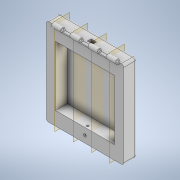
# Autodesk Inventor part: Bottom
Saved by Autodesk Inventor 2022 (Build 260153000, 153)
## iProperties
Created: 2022-03-05
Part Number: Bottom
Material: Generic
Document SubType Name: Modeling
Designer: Stump
Density: 1 g/cm^3
Appearance: Default
Author: Stump
Autodesk Inventor part; units mm, degrees
ref_plane "XZ Plane" through (0, 0, 0) normal (0, 1, 0) x (-1, 0, 0)
ref_plane "XY Plane" through (0, 0, 0) normal (0, 0, 1) x (1, 0, 0)
sketch "Sketch1" plane through (0, 0, 0) normal (0, 0, 1) x (1, 0, 0)
  line L0 (0, 0) -> (165.2524, 0)
  line L1 (165.2524, 0) -> (165.2524, 167.64)
  line L2 (165.2524, 167.64) -> (0, 167.64)
  line L3 (0, 167.64) -> (0, 0)
  line L4 (82.6262, 167.64) -> (82.6262, 205.74) construction
  line L5 (82.6262, 0) -> (82.6262, -38.1) construction
  line L6 (0, 83.82) -> (-25.4, 83.82) construction
  line L7 (165.2524, 83.82) -> (190.6524, 83.82) construction
  line L8 (-25.4981, -38.1) -> (190.6088, -38.1)
  line L9 (190.6088, -38.1) -> (190.6088, 205.74)
  line L10 (190.6088, 205.74) -> (-25.4981, 205.74)
  line L11 (-25.4981, 205.74) -> (-25.4981, -38.1)
  dimension "d0" = 165.2524
  dimension "d1" = 167.64
  dimension "d2" = 38.1
  dimension "d3" = 38.1
  dimension "d4" = 25.4
  dimension "d5" = 25.4
  constraints: 24 end point, 4 horizontal, 4 midpoint, 4 parallel, 2 perpendicular, 2 vertical
  measures "d0" distance of L2.end L1.end
  measures "d1" distance of L1.end L0.end
  measures "d2" distance of L4.start L4.end
  measures "d3" distance of L5.start L5.end
  measures "d4" distance of L6.start L6.end
  measures "d5" distance of L7.start L7.end
extrude "Extrusion1" add sketch "Sketch1" along normal blind 37.592
sketch "Sketch3" plane through (0, 0, 0) normal (0, 0, -1) x (-1, 0, 0)
  line L0 (6.0775, -8.2655) -> (-172.3593, -8.2655)
  line L1 (-172.3593, -8.2655) -> (-172.3593, 173.0886)
  line L2 (-172.3593, 173.0886) -> (6.0775, 173.0886)
  line L3 (6.0775, 173.0886) -> (6.0775, -8.2655)
  point P0 (0, 0)
  constraints: 8 end point, 2 parallel, 1 horizontal, 1 perpendicular
extrude "Extrusion3" add sketch "Sketch3" against normal blind 4.699
fillet "Fillet1" radius 6.35 8 edges at (-25.4981, 205.74, 18.796) (-25.4981, -38.1, 18.796) (190.6088, -38.1, 18.796) (190.6088, 205.74, 18.796) (190.6088, 83.82, 0) (82.5553, -38.1, 0) (-25.4981, 83.82, 0) (82.5553, 205.74, 0)
ref_plane "Work Plane1" through (0.254, 0, 0) normal (1, 0, 0) x (0, 1, 0)
sketch "Sketch4" plane through (0.254, 0, 0) normal (1, 0, 0) x (0, 1, 0)
  line L0 (205.74, 37.592) -> (217.17, 37.592) construction
  line L1 (217.17, 37.592) -> (217.17, 49.022) construction
  line L2 (217.17, 49.022) -> (205.74, 49.022) construction
  line L3 (205.74, 49.022) -> (205.74, 37.592) construction
  circle A0 centre (211.455, 43.307) radius 5.715
  circle A1 centre (211.455, 43.307) radius 3.302
  point P0 (0, 0)
  dimension "d14" = 11.43
  dimension "d15" = 11.43
  dimension "d16" = 6.604
  constraints: 8 end point, 3 perpendicular, 2 centre point, 1 coincident, 1 horizontal, 1 tangent
  measures "d14" distance of L0.start L0.end
  measures "d15" distance of L0.end L1.end
  measures "d16" diameter of A1
extrude "Extrusion4" add sketch "Sketch4" along normal blind 25.4
ref_plane "Work Plane2" through (51.308, 0, 0) normal (1, 0, 0) x (0, 1, 0)
sketch "Sketch5" plane through (51.308, 0, 0) normal (1, 0, 0) x (0, 1, 0)
  line L0 (205.74, 37.592) -> (217.17, 37.592) construction
  line L1 (217.17, 37.592) -> (217.17, 49.022) construction
  circle A0 centre (211.455, 43.307) radius 5.715
  circle A1 centre (211.455, 43.307) radius 3.302
  point P0 (0, 0)
  dimension "d20" = 11.43
  dimension "d21" = 11.43
  dimension "d22" = 6.604
  constraints: 4 end point, 2 centre point, 1 coincident, 1 horizontal, 1 perpendicular
  measures "d20" distance of L0.start L0.end
  measures "d21" distance of L0.end L1.end
  measures "d22" diameter of A1
extrude "Extrusion5" add sketch "Sketch5" along normal blind 25.4
ref_plane "Work Plane3" through (102.362, 0, 0) normal (1, 0, 0) x (0, 1, 0)
sketch "Sketch6" plane through (102.362, 0, 0) normal (1, 0, 0) x (0, 1, 0)
  line L0 (205.74, 37.592) -> (217.17, 37.592) construction
  line L1 (217.17, 37.592) -> (217.17, 49.022) construction
  circle A0 centre (211.455, 43.307) radius 5.715
  circle A1 centre (211.455, 43.307) radius 3.302
  point P0 (0, 0)
  dimension "d26" = 11.43
  dimension "d27" = 11.43
  dimension "d28" = 6.604
  constraints: 4 end point, 2 centre point, 1 coincident, 1 horizontal, 1 perpendicular
  measures "d26" distance of L0.start L0.end
  measures "d27" distance of L0.end L1.end
  measures "d28" diameter of A1
extrude "Extrusion6" add sketch "Sketch6" along normal blind 25.4
ref_plane "Work Plane4" through (153.416, 0, 0) normal (1, 0, 0) x (0, 1, 0)
sketch "Sketch7" plane through (153.416, 0, 0) normal (1, 0, 0) x (0, 1, 0)
  line L0 (205.74, 37.592) -> (217.17, 37.592) construction
  line L1 (217.17, 37.592) -> (217.17, 49.022) construction
  circle A0 centre (211.455, 43.307) radius 5.715
  circle A1 centre (211.455, 43.307) radius 3.302
  point P0 (0, 0)
  dimension "d32" = 11.43
  dimension "d33" = 11.43
  dimension "d34" = 6.604
  constraints: 4 end point, 2 centre point, 1 coincident, 1 horizontal, 1 perpendicular
  measures "d32" distance of L0.start L0.end
  measures "d33" distance of L0.end L1.end
  measures "d34" diameter of A1
extrude "Extrusion7" add sketch "Sketch7" along normal blind 25.4
sketch "Sketch9" plane through (0.254, 0, 0) normal (1, 0, 0) x (0, 1, 0)
  line L0 (199.39, 37.592) -> (199.39, 6.35) projected
  line L1 (207.6697, 43.307) -> (199.39, 43.307)
  line L2 (199.39, 43.307) -> (199.39, 35.6964)
  line L3 (199.39, 35.6964) -> (207.6697, 35.6964)
  line L4 (207.6697, 39.5017) -> (207.6697, 43.307)
  line L5 (199.39, 35.6964) -> (211.3726, 35.6964)
  line L6 (211.3726, 35.6964) -> (211.3726, 39.5017)
  line L7 (211.3726, 39.5017) -> (207.6697, 39.5017)
  line L8 (199.39, 39.5017) -> (199.39, 35.6964)
  point P0 (0, 0)
  point P1 (199.39, 37.592)
  constraints: 16 end point, 4 parallel, 2 horizontal, 2 perpendicular, 1 point on line
extrude "Extrusion8" add sketch "Sketch9" along normal blind 178.562
sketch "Sketch10" plane through (0.254, 211.3726, 35.6964) normal (0, 1, 0) x (1, 0, 0)
  line L0 (102.108, -1.8961) -> (102.108, -3.8053) projected
  line L1 (127.508, -1.8961) -> (102.108, -1.8961) projected
  line L2 (127.508, -3.8053) -> (127.508, -1.8961) projected
  line L3 (127.508, -3.8053) -> (153.162, -3.8053) projected
  line L4 (153.162, -1.8961) -> (153.162, -3.8053) projected
  line L5 (178.562, -1.8961) -> (153.162, -1.8961) projected
  line L6 (178.562, 0) -> (178.562, -1.8961) projected
  line L7 (0, 0) -> (178.562, 0) projected
  line L8 (0, 0) -> (0, -1.8961) projected
  line L9 (25.4, -1.8961) -> (0, -1.8961) projected
  line L10 (25.4, -3.8053) -> (25.4, -1.8961) projected
  line L11 (25.4, -3.8053) -> (51.054, -3.8053) projected
  line L12 (51.054, -1.8961) -> (51.054, -3.8053) projected
  line L13 (76.454, -1.8961) -> (51.054, -1.8961) projected
  line L14 (76.454, -3.8053) -> (76.454, -1.8961) projected
  line L15 (76.454, -3.8053) -> (102.108, -3.8053) projected
  line L16 (0, 0) -> (178.562, 0) projected
  line L17 (0, -7.6106) -> (178.562, -7.6106) projected
  line L18 (153.162, 0) -> (127.508, 0)
  line L19 (127.508, 0) -> (127.508, -7.6106)
  line L20 (127.508, -7.6106) -> (153.162, -7.6106)
  line L21 (153.162, -7.6106) -> (153.162, 0)
  line L22 (76.454, -7.6106) -> (102.108, -7.6106) projected
  line L23 (102.108, 0) -> (76.454, 0)
  line L24 (76.454, 0) -> (76.454, -7.6106)
  line L25 (76.454, -7.6106) -> (102.108, -7.6106)
  line L26 (102.108, -7.6106) -> (102.108, 0)
  line L27 (51.054, 0) -> (25.4, 0)
  line L28 (25.4, 0) -> (25.4, -7.6106)
  line L29 (25.4, -7.6106) -> (51.054, -7.6106)
  line L30 (51.054, -7.6106) -> (51.054, 0)
  point P0 (-0.254, 35.6964)
  point P1 (25.4, 0)
  point P2 (51.054, -7.6106)
  point P3 (51.054, -3.8053)
  point P4 (76.454, 0)
  constraints: 24 end point, 6 parallel, 5 point on line, 3 horizontal, 3 perpendicular
extrude "Extrusion9" cut sketch "Sketch10" against normal blind 5.715 contours L0 L15 L14 L24 L7 L26 | L26 L17 L24 L15 | L19 L7 L21 L4 L3 L2 | L3 L21 L17 L19 | L30 L12 L11 L10 L28 L7 | L17 L28 L11 L30
fillet "Fillet2" radius 6.35 4 edges at (166.116, 211.3726, 35.6964) (115.062, 211.3726, 35.6964) (64.008, 211.3726, 35.6964) (12.954, 211.3726, 35.6964)
fillet "Fillet3" radius 3.175 5 edges at (178.816, 199.39, 40.4495) (178.816, 202.565, 43.307) (89.535, 199.39, 43.307) (0.254, 202.565, 43.307) (0.254, 199.39, 40.4495)
sketch "Sketch11" plane through (0, 0, 37.592) normal (0, 0, 1) x (1, 0, 0)
  line L0 (0, 0) -> (0, 167.64) projected
  line L1 (165.2524, 0) -> (0, 0) projected
  line L2 (165.2524, 167.64) -> (165.2524, 0) projected
  line L3 (0, 167.64) -> (165.2524, 167.64) projected
  line L4 (0, 0) -> (0, 167.64) projected
  line L5 (165.2524, 0) -> (0, 0) construction
  line L6 (82.6262, 0) -> (82.5553, -38.1) construction
  line L7 (-19.1481, -38.1) -> (184.2588, -38.1) construction
  circle A0 centre (82.5908, -19.05) radius 3.7719
  dimension "d47" = 7.5438
  constraints: 3 midpoint, 2 end point, 1 centre point
  measures "d47" diameter of A0
extrude "Extrusion10" cut sketch "Sketch11" against normal blind 101.6 contours A0
sketch "Sketch13" plane through (0, 0, 0) normal (0, 0, -1) x (-1, 0, 0)
  circle A0 centre (-82.5908, -19.05) radius 3.7719 projected
  circle A1 centre (-82.5908, -19.05) radius 4.0259
  point P0 (0, 0)
  dimension "d50" = 8.0518
  constraints: 1 centre point, 1 coincident
  measures "d50" diameter of A1
extrude "Extrusion11" cut sketch "Sketch13" against normal blind 33.3502
sketch "Sketch14" plane through (0, 0, 37.592) normal (0, 1, 0) x (1, 0, 0)
  line L0 (86.3627, 4.2418) -> (78.8189, 4.2418) projected
  line L1 (82.5908, 4.2418) -> (82.5908, 10.5918)
  circle A0 centre (82.5908, 7.4168) radius 3.1152
  point P0 (0, 37.592)
  dimension "d53" = 6.35
  constraints: 2 end point, 2 midpoint, 1 centre point, 1 vertical
  measures "d53" distance of L1.start L1.end
extrude "Extrusion12" cut sketch "Sketch14" against normal blind 19.05
sketch "Sketch17" plane through (0, 167.64, 37.592) normal (0, -1, 0) x (1, 0, 0)
  line L0 (0.254, 0) -> (0.254, -1.8956) projected
  line L1 (0.254, -1.8956) -> (25.654, -1.8956) projected
  line L2 (25.654, -1.8956) -> (51.308, -1.8956) projected
  line L3 (51.308, -1.8956) -> (76.708, -1.8956) projected
  line L4 (76.708, -1.8956) -> (102.362, -1.8956) projected
  line L5 (102.362, -1.8956) -> (127.762, -1.8956) projected
  line L6 (127.762, -1.8956) -> (153.416, -1.8956) projected
  line L7 (153.416, -1.8956) -> (178.816, -1.8956) projected
  line L8 (178.816, -1.8956) -> (178.816, 0) projected
  line L9 (184.2588, 0) -> (178.816, 0) projected
  line L10 (184.2588, -31.242) -> (184.2588, 0) projected
  line L11 (-19.1481, -31.242) -> (184.2588, -31.242) projected
  line L12 (-19.1481, 0) -> (-19.1481, -31.242) projected
  line L13 (0.254, 0) -> (-19.1481, 0) projected
  line L14 (-19.1481, -31.242) -> (184.2588, -31.242) projected
  line L15 (89.535, -31.242) -> (89.535, -17.5006)
  line L16 (89.535, -17.5006) -> (82.0801, -17.5006)
  line L17 (82.0801, -17.5006) -> (82.0801, -7.0104)
  line L18 (82.0801, -7.0104) -> (97.3201, -7.0104)
  line L19 (97.3201, -7.0104) -> (97.3201, -17.5006)
  line L20 (97.3201, -17.5006) -> (82.0801, -17.5006)
  line L21 (82.0801, -17.5006) -> (82.0801, -7.0104)
  point P0 (0, -37.592)
  dimension "d63" = 13.7414
  dimension "d64" = 7.4549
  dimension "d65" = 10.4902
  dimension "d66" = 15.24
  constraints: 14 end point, 3 parallel, 3 perpendicular, 1 horizontal, 1 point on line
  measures "d63" distance of L15.start L15.end
  measures "d64" distance of L15.end L16.end
  measures "d65" distance of L16.end L17.end
  measures "d66" distance of L19.end L20.end
extrude "Extrusion14" cut sketch "Sketch17" against normal blind 76.2 contours L16 L17 L18 L19 L20
sketch "Sketch18" plane through (0, 0, 0) normal (0, 0, -1) x (-1, 0, 0)
  circle A0 centre (-82.5908, -19.05) radius 3.7719 projected
  circle A1 centre (-82.5908, -19.05) radius 6.35
  point P0 (0, 0)
  dimension "d69" = 12.7
  constraints: 1 centre point, 1 coincident
  measures "d69" diameter of A1
extrude "Extrusion15" add sketch "Sketch18" against normal blind 2.54 contours A0 | A1
body "Solid1"
